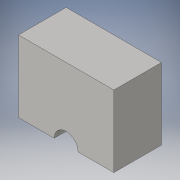
# Autodesk Inventor part: StandAloneLift
Saved by Autodesk Inventor 2016 SP1 (Build 200210100, 210)
## iProperties
Created: 2016-02-05
Part Number: StandAloneLift
Material: Generic
Document SubType Name: Modeling
Designer: steele
Density: 1 g/cm^3
Appearance: Default
Author: steele
Autodesk Inventor part; units mm, degrees
ref_plane "YZ Plane" through (0, 0, 0) normal (1, 0, 0) x (0, 1, 0)
ref_plane "XZ Plane" through (0, 0, 0) normal (0, 1, 0) x (-1, 0, 0)
ref_plane "XY Plane" through (0, 0, 0) normal (0, 0, 1) x (1, 0, 0)
sketch "Sketch1" plane through (0, 0, 0) normal (0, 1, 0) x (-1, 0, 0)
  line L0 (25.4, 12.7) -> (-25.4, 12.7)
  line L1 (-25.4, 12.7) -> (-25.4, -12.7)
  line L2 (-25.4, -12.7) -> (25.4, -12.7)
  line L3 (25.4, -12.7) -> (25.4, 12.7)
  line L4 (25.4, 12.7) -> (-25.4, -12.7) construction
  line L5 (-25.4, 12.7) -> (25.4, -12.7) construction
  point P0 (0, 0)
  dimension "d0" = 25.4
  dimension "d1" = 50.8
  constraints: 12 end point, 2 midpoint, 2 parallel, 1 horizontal, 1 perpendicular
  measures "d0" distance of L0.end L1.end
  measures "d1" distance of L1.end L2.end
extrude "Extrusion1" add sketch "Sketch1" against normal blind 38.1
sketch "Sketch2" plane through (-25.4, 0, 12.7) normal (0, 0, 1) x (1, 0, 0)
  line L0 (50.8, -38.1) -> (0, -38.1) projected
  circle A0 centre (25.4, -38.1) radius 6.35
  point P0 (25.4, 0)
  dimension "d4" = 12.7
  constraints: 1 centre point, 1 midpoint
  measures "d4" diameter of A0
extrude "Extrusion2" cut sketch "Sketch2" against normal through all
body "Solid1"
